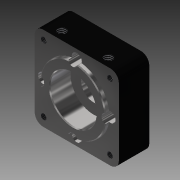
# Autodesk Inventor part: P80 Motor Block
Saved by Autodesk Inventor 2013 (Build 170138000, 138)
## iProperties
Created: 2013-02-10
Part Number: P80 Motor Block
Material: Steel
Document SubType Name: Modeling
Designer: Moses
Density: 7.85 g/cm^3
Mass: 588.644 g
Surface Area: 185.544 cm^2
Volume: 74.9865 cm^3
Author: Moses
Autodesk Inventor part; units mm, degrees
ref_plane "YZ Plane" through (0, 0, 0) normal (1, 0, 0) x (0, 1, 0)
ref_plane "XZ Plane" through (0, 0, 0) normal (0, 1, 0) x (-1, 0, 0)
ref_plane "XY Plane" through (0, 0, 0) normal (0, 0, 1) x (1, 0, 0)
sketch "Sketch1" plane through (0, 0, 0) normal (0, 0, 1) x (1, 0, 0)
  circle A0 centre (0, 0) radius 9.525
  circle A1 centre (0, 0) radius 17.4625
  line L0 (-31.75, 31.75) -> (31.75, 31.75)
  line L1 (31.75, 31.75) -> (31.75, -31.75)
  line L2 (31.75, -31.75) -> (-31.75, -31.75)
  line L3 (-31.75, -31.75) -> (-31.75, 31.75)
  line L4 (-31.75, 0) -> (31.75, 0) construction
  line L5 (0, 31.75) -> (0, -31.75) construction
  circle A2 centre (0, 25.4) radius 2.3495
  circle A3 centre (-25.4, 0) radius 2.3495
  circle A4 centre (25.4, 0) radius 2.3495
  circle A5 centre (0, -25.4) radius 2.3495
  line L6 (-27.0002, 27.0002) -> (27.0002, 27.0002) construction
  line L7 (27.0002, 27.0002) -> (27.0002, -27.0002) construction
  line L8 (27.0002, -27.0002) -> (-27.0002, -27.0002) construction
  line L9 (-27.0002, -27.0002) -> (-27.0002, 27.0002) construction
  circle A6 centre (-25.0002, 25.0002) radius 2 construction
  circle A7 centre (25.0002, 25.0002) radius 2 construction
  circle A8 centre (25.0002, -25.0002) radius 2 construction
  circle A9 centre (-25.0002, -25.0002) radius 2 construction
  circle A10 centre (0, 25.4) radius 3.81
  circle A11 centre (25.4, 0) radius 3.81
  circle A12 centre (-25.4, 0) radius 3.81
  circle A13 centre (0, -25.4) radius 3.81
  arc A14 (-24.3637, -3.6664) -> (-3.6664, -24.3637) centre (0, 0) ccw
  arc A15 (3.6664, -24.3637) -> (24.3637, -3.6664) centre (0, 0) ccw
  arc A16 (24.3637, 3.6664) -> (3.6664, 24.3637) centre (0, 0) ccw
  arc A17 (-3.6664, 24.3637) -> (-24.3637, 3.6664) centre (0, 0) ccw
  circle A18 centre (-25.0002, 25.0002) radius 2.1209
  circle A19 centre (25.0002, 25.0002) radius 2.1209
  circle A20 centre (25.0002, -25.0002) radius 2.1209
  circle A21 centre (-25.0002, -25.0002) radius 2.1209
  point P0 (0, 27.0002)
  point P1 (-27.0002, 0)
  dimension "d0" = 19.05
  dimension "d2" = 63.5
  dimension "d3" = 63.5
  dimension "d4" = 4.699
  dimension "d6" = 25.4
  dimension "d7" = 25.4
  dimension "d8" = 25.4
  dimension "d9" = 25.4
  dimension "d10" = 34.925
  dimension "d13" = 54.0004
  dimension "d14" = 54.0004
  dimension "d15" = 4
  dimension "d16" = 24.638
  dimension "d17" = 7.62
  dimension "d26" = 4.2418
  constraints: 22 centre point, 20 end point, 16 point on circle, 15 equal radius, 12 coincident, 8 tangent, 7 midpoint, 6 point on line, 4 parallel, 2 horizontal, 2 perpendicular
  measures "d0" diameter of A0
  measures "d2" distance of L0.start L0.end
  measures "d3" distance of L0.end L1.end
  measures "d4" diameter of A2
  measures "d6" distance from line of L4 A2.centre
  measures "d7" distance from line of A5.centre L4
  measures "d8" distance from line of L5 A3.centre
  measures "d9" distance from line of A4.centre L5
  measures "d10" diameter of A1
  measures "d13" distance of L6.start L6.end
  measures "d14" distance of L6.end L7.end
  measures "d15" diameter of A6
  measures "d16" radius of A17
  measures "d17" diameter of A10
  measures "d26" diameter of A18
extrude "Extrusion1" add sketch "Sketch1" against normal blind 22.9108 contours A1 | L0 L1 L2 L3 | A10 | A10 A16 A11 A15 A13 A14 A12 A17 | A12 | A11 | A13
extrude "Extrusion2" cut sketch "Sketch1" against normal blind 12.7 contours A1 | A10 | A12 | A11 | A13
extrude "Extrusion3" add sketch "Sketch1" along normal blind 3 contours A10 A16 A11 A15 A13 A14 A12 A17
fillet "Fillet1" radius 6.35 4 edges at (-31.75, 31.75, -11.4554) (31.75, 31.75, -11.4554) (-31.75, -31.75, -11.4554) (31.75, -31.75, -11.4554)
chamfer "Chamfer1" distance 0.635 angle 45 6 edges at (-17.4625, 0, 3) (-9.525, 0, -22.9108) (17.4217, -17.4217, 3) (-17.4217, -17.4217, 3) (-17.4217, 17.4217, 3) (17.4217, 17.4217, 3)
thread "Thread1" size "10-32 UNF" class "2B" standard "ANSI Unified Screw Threads" full length
thread "Thread2" size "10-32 UNF" class "2B" standard "ANSI Unified Screw Threads" full length
thread "Thread3" size "10-32 UNF" class "2B" standard "ANSI Unified Screw Threads" full length
thread "Thread4" size "10-32 UNF" class "2B" standard "ANSI Unified Screw Threads" full length
sketch "Sketch2" plane through (-25.4, -31.75, 0) normal (0, -1, 0) x (1, 0, 0)
  line L0 (50.8, -22.9108) -> (0, -22.9108) projected
  line L1 (7.8994, -6.35) -> (42.9006, -6.35) construction
  circle A0 centre (7.8994, -6.35) radius 3.175
  circle A1 centre (42.9006, -6.35) radius 3.175
  line L2 (25.4, -22.9108) -> (25.4, 0) construction
  point P0 (25.4, -6.35)
  dimension "d35" = 35.0012
  dimension "d37" = 6.35
  dimension "d38" = 16.5608
  constraints: 4 end point, 2 centre point, 2 coincident, 2 midpoint, 1 equal radius, 1 perpendicular, 1 point on line
  measures "d35" distance of L1.start L1.end
  measures "d37" diameter of A0
  measures "d38" distance between parallel lines of L0 L1
extrude "Extrusion4" cut sketch "Sketch2" against normal blind 12.7
sketch "Sketch3" plane through (-25.4, 31.75, 0) normal (0, 1, 0) x (1, 0, 0)
  line L0 (0, 22.9108) -> (50.8, 22.9108) projected
  line L1 (0, 0) -> (50.8, 0) projected
  line L2 (7.8994, 6.35) -> (42.9006, 6.35) construction
  line L3 (25.4, 22.9108) -> (25.4, 0) construction
  circle A0 centre (7.8994, 6.35) radius 3.175
  circle A1 centre (42.9006, 6.35) radius 3.175
  point P0 (25.4, 6.35)
  dimension "d41" = 6.35
  dimension "d43" = 16.5608
  dimension "d44" = 35.0012
  constraints: 4 end point, 2 centre point, 2 coincident, 2 midpoint, 1 equal radius, 1 parallel, 1 perpendicular, 1 point on line
  measures "d41" diameter of A0
  measures "d43" distance between parallel lines of L0 L2
  measures "d44" distance of L2.start L2.end
extrude "Extrusion5" cut sketch "Sketch3" against normal blind 12.7
thread "Thread5" size "1/4-20 UNC" class "2B" standard "ANSI Unified Screw Threads" full length
thread "Thread6" size "1/4-20 UNC" class "2B" standard "ANSI Unified Screw Threads" full length
thread "Thread7" size "1/4-20 UNC" class "2B" standard "ANSI Unified Screw Threads" full length
thread "Thread8" size "1/4-20 UNC" class "2B" standard "ANSI Unified Screw Threads" full length
body "Solid1"
